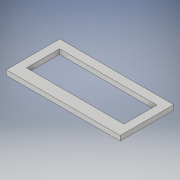
# Autodesk Inventor part: painel lcd
Saved by Autodesk Inventor 2019.4 (Build 234330000, 330)
## iProperties
Created: 2019-11-13
Part Number: painel lcd
Material: Genérico
Document SubType Name: Modeling
Designer: natha
Density: 1 g/cm^3
Appearance: Padrão
Author: natha
Autodesk Inventor part; units mm, degrees
ref_plane "YZ Plane" through (0, 0, 0) normal (1, 0, 0) x (0, 1, 0)
ref_plane "XZ Plane" through (0, 0, 0) normal (0, 1, 0) x (-1, 0, 0)
ref_plane "XY Plane" through (0, 0, 0) normal (0, 0, 1) x (1, 0, 0)
sketch "Esboço1" plane through (0, 0, 0) normal (0, 1, 0) x (-1, 0, 0)
  circle A0 centre (89.65, -41.2701) radius 1.5
  circle A1 centre (89.65, -10.2701) radius 1.5
  circle A2 centre (14.65, -10.2701) radius 1.5
  circle A3 centre (14.65, -41.2701) radius 1.5
  line L0 (14.65, -10.2701) -> (10.65, -10.2701) construction
  line L1 (10.65, -10.2701) -> (10.65, -6.2701) construction
  line L2 (10.65, -6.2701) -> (93.65, -6.2701)
  line L3 (93.65, -6.2701) -> (93.65, -45.2701)
  line L4 (93.65, -45.2701) -> (10.65, -45.2701)
  line L5 (10.65, -45.2701) -> (10.65, -6.2701)
  line L6 (87.5, -38.8701) -> (87.5, -14.8701) construction
  line L7 (87.5, -14.8701) -> (16.5, -14.8701) construction
  line L8 (16.5, -14.8701) -> (16.5, -38.8701) construction
  line L9 (16.5, -38.8701) -> (87.5, -38.8701) construction
  line L10 (87.5, -14.8701) -> (88.5, -14.8701) construction
  line L11 (88.5, -14.8701) -> (88.5, -13.8701) construction
  line L12 (88.5, -13.8701) -> (87.5, -13.8701) construction
  line L13 (87.5, -13.8701) -> (87.5, -14.8701) construction
  circle A4 centre (14.65, -10.2701) radius 2.85
  circle A5 centre (14.65, -41.2701) radius 2.85
  circle A6 centre (89.65, -41.2701) radius 2.85
  circle A7 centre (89.65, -10.2701) radius 2.85
  line L14 (16.5, -14.8701) -> (87.5, -14.8701)
  line L15 (87.5, -14.8701) -> (87.5, -38.8701)
  line L16 (87.5, -38.8701) -> (16.5, -38.8701)
  line L17 (16.5, -38.8701) -> (16.5, -14.8701)
  point P0 (0, 0)
  dimension "d0" = 4
  dimension "d1" = 4
  dimension "d2" = 4
  dimension "d3" = 4
  dimension "d4" = 4
  dimension "d5" = 4
  dimension "d6" = 4
  dimension "d7" = 4
  dimension "d8" = 1
  dimension "d9" = 1
  dimension "d10" = 5.7
  dimension "d11" = 5.7
  dimension "d12" = 5.7
  dimension "d13" = 5.7
  constraints: 36 end point, 8 centre point, 6 horizontal, 6 parallel, 4 coincident, 4 perpendicular, 2 vertical, 4 other
  measures "d0" distance of L0.start L0.end
  measures "d1" distance of L0.end L2.start
  measures "d2" distance from line of L5 A3.centre
  measures "d3" distance from line of L4 A3.centre
  measures "d4" distance from line of A0.centre L3
  measures "d5" distance from line of L4 A0.centre
  measures "d6" distance from line of L2 A1.centre
  measures "d7" distance from line of L3 A1.centre
  measures "d8" distance of L11.end L13.start
  measures "d9" distance of L11.start L11.end
  measures "d10" diameter of A4
  measures "d11" diameter of A5
  measures "d12" diameter of A6
  measures "d13" diameter of A7
extrude "Extrusão1" add sketch "Esboço1" along normal blind 2.5 contours L2 L3 L4 L5
sketch "Esboço2" plane through (0, 2.5, 0) normal (0, 1, 0) x (1, 0, 0)
  line L0 (-93.65, 6.2701) -> (-10.65, 6.2701) projected
  line L1 (-93.65, 45.2701) -> (-93.65, 6.2701) projected
  line L2 (-10.65, 6.2701) -> (-93.65, 6.2701)
  line L3 (-93.65, 6.2701) -> (-93.65, 45.2701)
  line L4 (-93.65, 45.2701) -> (-10.65, 45.2701)
  line L5 (-10.65, 45.2701) -> (-10.65, 6.2701)
  line L6 (-87.5, 14.8701) -> (-87.5, 38.8701) projected
  line L7 (-16.5, 14.8701) -> (-87.5, 14.8701) projected
  line L8 (-87.5, 38.8701) -> (-16.5, 38.8701)
  line L9 (-16.5, 38.8701) -> (-16.5, 14.8701)
  line L10 (-16.5, 14.8701) -> (-87.5, 14.8701)
  line L11 (-87.5, 14.8701) -> (-87.5, 38.8701)
  point P0 (0, 0)
  constraints: 16 end point, 4 parallel, 2 horizontal, 2 perpendicular
extrude "Extrusão2" add sketch "Esboço2" along normal blind 1
